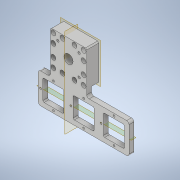
# Autodesk Inventor part: 30_XY_Sample_arm_UC2_Adapter_v3
Saved by Autodesk Inventor 2022.3 (Build 263350000, 350)
## iProperties
Created: 2020-12-29
Part Number: 30_XY_Sample_arm_UC2_Adapter_v3
Material: Generic
Document SubType Name: Modeling
Designer: diederichbenedict
Density: 1 g/cm^3
Appearance: Default
Author: diederichbenedict
Autodesk Inventor part; units mm, degrees
ref_plane "YZ Plane" through (0, 0, 0) normal (1, 0, 0) x (0, 1, 0)
ref_plane "XZ Plane" through (0, 0, 0) normal (0, 1, 0) x (-1, 0, 0)
ref_plane "XY Plane" through (0, 0, 0) normal (0, 0, 1) x (1, 0, 0)
ref_plane "Work Plane1" through (0, 0, 0) normal (0, 0, 1) x (1, 0, 0)
sketch "Sketch1" plane through (0, 0, 0) normal (0, 0, 1) x (1, 0, 0)
  circle A0 centre (-10, -25) radius 1.45 projected
  circle A1 centre (-10, 25) radius 1.45 projected
  circle A2 centre (10, 25) radius 1.45 projected
  circle A3 centre (10, -25) radius 1.45 projected
  circle A4 centre (-25, 25) radius 2.325 projected
  circle A5 centre (25, -25) radius 2.325 projected
  circle A6 centre (-25, -25) radius 2.325 projected
  circle A7 centre (25, 25) radius 2.325 projected
  line L0 (28, 30) -> (30, 28) projected
  line L1 (28, 30) -> (-28, 30) projected
  line L2 (-30, 28) -> (-28, 30) projected
  line L3 (-30, 28) -> (-30, -28) projected
  line L4 (-28, -30) -> (-30, -28) projected
  line L5 (-28, -30) -> (28, -30) projected
  line L6 (30, -28) -> (28, -30) projected
  line L7 (30, -28) -> (30, 28) projected
  circle A8 centre (-17.5, -17.5) radius 1.95 projected
  circle A9 centre (17.5, 17.5) radius 1.95 projected
  circle A10 centre (17.5, -17.5) radius 1.95 projected
  circle A11 centre (-17.5, 17.5) radius 1.95 projected
  circle A12 centre (0, 0) radius 7.5 projected
  circle A13 centre (-25.33, -75.26) radius 6.15 projected
  circle A14 centre (25, -10) radius 1.45 projected
  circle A15 centre (-25, -10) radius 1.45 projected
  circle A16 centre (-25, 10) radius 1.45 projected
  circle A17 centre (25, 10) radius 1.45 projected
  point P0 (0, 0)
extrude "Extrusion1" add sketch "Sketch1" along normal blind 12 contours L0 L7 L6 L5 L4 L3 L2 L1
sketch "Sketch2" plane through (0, 0, 12) normal (0, 0, 1) x (1, 0, 0)
  circle A0 centre (0, 0) radius 7.5 projected
  circle A1 centre (25, 10) radius 1.45 projected
  circle A2 centre (-25, 10) radius 1.45 projected
  circle A3 centre (-25, -10) radius 1.45 projected
  circle A4 centre (25, -10) radius 1.45 projected
  circle A5 centre (10, -25) radius 1.45 projected
  circle A6 centre (10, 25) radius 1.45 projected
  circle A7 centre (-10, 25) radius 1.45 projected
  circle A8 centre (-10, -25) radius 1.45 projected
  line L0 (-28, -30) -> (28, -30) projected
  line L1 (28, -30) -> (30, -28) projected
  line L2 (30, -28) -> (30, 28) projected
  line L3 (30, 28) -> (28, 30) projected
  line L4 (28, 30) -> (-28, 30) projected
  line L5 (30, -28) -> (30, 28) projected
  line L6 (30, -30) -> (28, -30)
  line L7 (18, -90) -> (30, -90)
  line L8 (30, -90) -> (30, -88) construction
  line L9 (30, 28) -> (30, -28) projected
  line L10 (30, -30) -> (30, -28)
  line L11 (30, -28) -> (28, -30)
  line L12 (-28, 30) -> (-30, 28) projected
  line L13 (-30, 28) -> (-30, -28) projected
  line L14 (-30, -28) -> (-28, -30) projected
  line L15 (-30, -30) -> (-28, -30)
  line L16 (-18, -90) -> (-30, -90)
  line L17 (-30, -30) -> (-30, -28)
  line L18 (-30, -28) -> (-28, -30)
  line L19 (-28, -30) -> (-30, -30)
  line L20 (28, -30) -> (30, -28) projected
  line L21 (28, -30) -> (30, -30)
  line L22 (30, -30) -> (30, -28)
  line L23 (30, -28) -> (28, -30)
  circle A9 centre (-17.5, 17.5) radius 1.95 projected
  circle A10 centre (-25, 25) radius 2.325 projected
  circle A11 centre (25, 25) radius 2.325 projected
  circle A12 centre (17.5, 17.5) radius 1.95 projected
  circle A13 centre (17.5, -17.5) radius 1.95 projected
  circle A14 centre (25, -25) radius 2.325 projected
  circle A15 centre (-25, -25) radius 2.325 projected
  line L24 (-18, -90) -> (18, -90)
  line L25 (18, -30) -> (-18, -30)
  line L26 (-50, -90) -> (-32, -90)
  line L27 (50, -90) -> (50, -40) construction
  line L28 (50, -40) -> (30, -40)
  line L29 (-50, -40) -> (-50, -90)
  line L30 (50, -40) -> (98, -40)
  line L31 (100, -40) -> (100, -42)
  line L32 (100, -90) -> (50, -90)
  line L33 (50, -90) -> (50, -40) construction
  line L34 (-30, -40) -> (-30, -30)
  line L35 (-30, -90) -> (-18, -90)
  line L36 (-18, -90) -> (18, -90)
  line L37 (18, -90) -> (30, -90)
  line L38 (30, -90) -> (32, -90)
  line L39 (32, -90) -> (50, -90)
  line L40 (100, -42) -> (100, -90)
  line L41 (98, -40) -> (100, -40)
  line L42 (30, -40) -> (18, -40)
  line L43 (-30, -90) -> (-30, -88) construction
  line L44 (-30, -40) -> (-50, -40)
  line L45 (-30, -88) -> (-30, -40) construction
  line L46 (-32, -90) -> (-30, -90)
  line L47 (18, -40) -> (-18, -40)
  line L48 (-18, -40) -> (-30, -40)
  line L49 (30, -40) -> (30, -30)
  line L50 (30, -88) -> (30, -40) construction
  line L51 (28, -30) -> (18, -30)
  line L52 (-28, -30) -> (-18, -30)
  line L53 (30, -28) -> (30, -30)
  line L54 (30, -28) -> (30, -30)
  line L55 (28, -30) -> (30, -30)
  line L56 (28, -30) -> (30, -28)
  point P0 (0, 0)
  point P1 (-24.2387, -104)
  point P2 (18, -80)
  point P3 (0, -40)
  point P4 (0, -30)
  dimension "d78" = 60
  dimension "d79" = 50
  dimension "d80" = 10
  dimension "d81" = 100
  dimension "d82" = 50
  constraints: 92 end point, 45 parallel, 14 horizontal, 13 collinear, 12 perpendicular, 12 point on line, 2 vertical, 1 midpoint, 1 vertical alignment
  measures "d78" distance between parallel lines of L0 L24
  measures "d79" distance between parallel lines of L26 L28
  measures "d80" distance from line of L28 L6.start
  measures "d81" distance between parallel lines of L27 L29
  measures "d82" distance between parallel lines of L31 L27
extrude "Extrusion2" add sketch "Sketch2" along normal blind 8
fillet "Fillet1" radius 4 6 edges at (-50, -40, 16) (-50, -90, 16) (100, -90, 16) (100, -40, 16) (30, -40, 16) (-30, -40, 16)
ref_plane "Work Plane2" through (-6, -91, 19) normal (1, 0, 0) x (0, 0, -1)
sketch "Sketch7" plane through (0, 0, 20) normal (0, 0, 1) x (1, 0, 0)
  circle A0 centre (10, -25) radius 1.45 projected
  circle A1 centre (-10, -25) radius 1.45 projected
  circle A2 centre (-25, -10) radius 1.45 projected
  circle A3 centre (-25, 10) radius 1.45 projected
  circle A4 centre (-10, 25) radius 1.45 projected
  circle A5 centre (10, 25) radius 1.45 projected
  circle A6 centre (25, 10) radius 1.45 projected
  circle A7 centre (25, -10) radius 1.45 projected
  circle A8 centre (-25, 25) radius 2.325 projected
  circle A9 centre (25, 25) radius 2.325 projected
  circle A10 centre (25, -25) radius 2.325 projected
  circle A11 centre (-25, -25) radius 2.325 projected
  point P0 (0, 0)
hole "Hole1" at (-25, -10, 20) at (-25, 10, 20) at (-10, 25, 20) at (10, 25, 20) at (25, 10, 20) at (25, -10, 20) at (10, -25, 20) at (-10, -25, 20) at (-25, 25, 20) at (-25, -25, 20) at (25, -25, 20) at (25, 25, 20) direction (0, 0, -1) diameter 3.2 end through all counterbore diameter 8 counterbore depth 10
sketch "Sketch12" plane through (0, 0, 12) normal (0, 0, -1) x (-1, 0, 0)
  line L0 (30.1502, -90.0017) -> (48, -90.0017)
  arc A0 (48, -90.0017) -> (50, -88.0017) centre (48, -88.0017) ccw
  line L1 (50, -70.0017) -> (50, -88.0017)
  arc A1 (50, -41.8579) -> (48, -39.8579) centre (48, -41.8579) ccw
  line L2 (48, -39.8579) -> (30, -39.8579)
  arc A2 (2, -40.0017) -> (0, -42.0017) centre (2, -42.0017) ccw
  line L3 (0, -59.8506) -> (0, -42.0017)
  arc A3 (0, -88.0017) -> (2, -90.0017) centre (2, -88.0017) ccw
  line L4 (9.561, -82.3) -> (40.161, -82.3)
  arc A4 (7.561, -80.3) -> (9.561, -82.3) centre (9.561, -80.3) ccw
  line L5 (7.561, -80.3) -> (7.561, -49.7)
  arc A5 (9.561, -47.7) -> (7.561, -49.7) centre (9.561, -49.7) ccw
  line L6 (40.161, -47.7) -> (9.561, -47.7)
  arc A6 (42.161, -49.7) -> (40.161, -47.7) centre (40.161, -49.7) ccw
  line L7 (42.161, -49.7) -> (42.161, -80.3)
  arc A7 (40.161, -82.3) -> (42.161, -80.3) centre (40.161, -80.3) ccw
  circle A8 centre (46.161, -65) radius 3.89
  circle A9 centre (24.761, -43.7) radius 2.9259
  line L8 (50, -70.0017) -> (50.8263, -70.0017)
  arc A10 (51.3, -70.3417) -> (50.8263, -70.0017) centre (50.8263, -70.5017) ccw
  arc A11 (51.3, -70.3417) -> (53.2596, -71.9417) centre (53.2596, -69.9417) ccw
  line L9 (53.2596, -71.9417) -> (53.4, -71.9417)
  arc A12 (53.4, -71.9417) -> (55.4, -69.9417) centre (53.4, -69.9417) ccw
  line L10 (55.4, -69.9417) -> (55.4, -60.0583)
  arc A13 (55.4, -60.0583) -> (53.4, -58.0583) centre (53.4, -60.0583) ccw
  line L11 (53.4, -58.0583) -> (53.2596, -58.0583)
  arc A14 (53.2596, -58.0583) -> (51.3, -59.6583) centre (53.2596, -60.0583) ccw
  arc A15 (50.8263, -59.9983) -> (51.3, -59.6583) centre (50.8263, -59.4983) ccw
  line L12 (50.8263, -59.9983) -> (50, -59.9983)
  line L13 (50, -41.8579) -> (50, -59.9983)
  line L14 (30, -39.8579) -> (30, -39.1754)
  arc A16 (30.34, -38.7017) -> (30, -39.1754) centre (30.5, -39.1754) ccw
  arc A17 (30.34, -38.7017) -> (31.94, -36.7421) centre (29.94, -36.7421) ccw
  line L15 (31.94, -36.7421) -> (31.94, -36.6017)
  arc A18 (31.94, -36.6017) -> (29.94, -34.6017) centre (29.94, -36.6017) ccw
  line L16 (29.94, -34.6017) -> (20.06, -34.6017)
  arc A19 (20.06, -34.6017) -> (18.06, -36.6017) centre (20.06, -36.6017) ccw
  line L17 (18.06, -36.6017) -> (18.06, -36.7421)
  arc A20 (18.06, -36.7421) -> (19.66, -38.7017) centre (20.06, -36.7421) ccw
  arc A21 (20, -39.1754) -> (19.66, -38.7017) centre (19.5, -39.1754) ccw
  line L18 (20, -39.1754) -> (20, -40.0017)
  line L19 (20, -40.0017) -> (2, -40.0017)
  line L20 (19.8489, -90.0017) -> (19.8491, -89.2759)
  arc A22 (19.8491, -89.2759) -> (19.6194, -88.9515) centre (19.5001, -89.2795) ccw
  arc A23 (17.9053, -86.8424) -> (19.6194, -88.9515) centre (20.06, -86.8424) ccw
  line L21 (17.9053, -86.8424) -> (17.9053, -86.7026)
  arc A24 (20.0566, -84.5515) -> (17.9053, -86.7026) centre (20.0565, -86.7026) ccw
  line L22 (20.0566, -84.5515) -> (29.94, -84.552)
  arc A25 (32.09, -86.7021) -> (29.94, -84.552) centre (29.94, -86.702) ccw
  line L23 (32.09, -86.7021) -> (32.09, -86.8424)
  arc A26 (30.38, -88.9468) -> (32.09, -86.8424) centre (29.9401, -86.8423) ccw
  arc A27 (30.38, -88.9468) -> (30.1502, -89.2756) centre (30.5004, -89.2756) ccw
  line L24 (30.1502, -89.2756) -> (30.1502, -90.0017)
  line L25 (0, -59.8506) -> (0.7258, -59.8508)
  arc A28 (0.7258, -59.8508) -> (1.0502, -59.6211) centre (0.7222, -59.5018) ccw
  arc A29 (3.1593, -57.907) -> (1.0502, -59.6211) centre (3.1593, -60.0617) ccw
  line L26 (3.1593, -57.907) -> (3.2991, -57.907)
  arc A30 (5.4502, -60.0583) -> (3.2991, -57.907) centre (3.2991, -60.0582) ccw
  line L27 (5.4502, -60.0583) -> (5.4497, -69.9417)
  arc A31 (3.2996, -72.0917) -> (5.4497, -69.9417) centre (3.2997, -69.9417) ccw
  line L28 (3.2996, -72.0917) -> (3.1593, -72.0917)
  arc A32 (1.0549, -70.3817) -> (3.1593, -72.0917) centre (3.1594, -69.9418) ccw
  arc A33 (1.0549, -70.3817) -> (0.7261, -70.1519) centre (0.7261, -70.5021) ccw
  line L29 (0.7261, -70.1519) -> (0, -70.152)
  line L30 (0, -88.0017) -> (0, -70.152)
  line L31 (2, -90.0017) -> (19.8489, -90.0017)
  line L32 (50, -44) -> (50, -86) projected
  line L33 (-0.1817, -64.8173) -> (24.3267, -108.886) construction
  line L34 (-100, -86) -> (-100, -44) projected
  line L35 (50, -44) -> (50, -86) projected
  point P0 (24.211, -65)
  point P1 (50, -65)
  point P2 (55.4, -65)
  point P3 (42.161, -65)
  point P4 (50, -65)
  point P5 (5.45, -65)
  point P6 (50, -65)
  point P7 (7.561, -65)
  point P8 (50, -65)
  point P9 (50, -65)
  dimension "d106" = 7.78
  dimension "d107" = 4
  dimension "d108" = 21.4
  dimension "d109" = 4
  constraints: 66 end point, 64 point on circle, 34 centre point, 7 horizontal alignment, 5 midpoint, 1 coincident, 1 collinear, 5 other
  measures "d106" diameter of A8
  measures "d107" distance from line of A8.centre L7
  measures "d108" horizontal distance of A9.centre A8.centre
  measures "d109" distance from line of L6 A9.centre
hole "Hole2" at (-46.161, -65, 12) at (-24.761, -43.7, 12) direction (0, 0, 1) diameter 3.2 end through all
pattern_linear "Rectangular Pattern1" count 3 spacing 50 along (1, 0, 0) of "Hole2"
sketch "Sketch15" plane through (0, 0, 12) normal (0, 0, -1) x (-1, 0, 0)
  line L0 (50, -40) -> (0, -40)
  line L1 (-100, -40) -> (-100, -90)
  line L2 (-100, -90) -> (-50, -90)
  line L3 (50, -90) -> (50, -40)
  line L4 (46, -90) -> (-96, -90) projected
  line L5 (-50, -40) -> (-50, -90)
  line L6 (50, -44) -> (50, -86) projected
  arc A0 (50, -44) -> (46, -40) centre (46, -44) ccw projected
  line L7 (34, -40) -> (46, -40) projected
  arc A1 (30, -36) -> (34, -40) centre (34, -36) ccw projected
  line L8 (30, -28) -> (30, -36) projected
  arc A2 (46, -90) -> (50, -86) centre (46, -86) ccw projected
  line L9 (46, -90) -> (-96, -90) projected
  arc A3 (-100, -86) -> (-96, -90) centre (-96, -86) ccw projected
  line L10 (-100, -86) -> (-100, -44) projected
  arc A4 (-96, -40) -> (-100, -44) centre (-96, -44) ccw projected
  line L11 (-96, -40) -> (-34, -40) projected
  arc A5 (-34, -40) -> (-30, -36) centre (-34, -36) ccw projected
  line L12 (-30, -36) -> (-30, -28) projected
  line L13 (0, -40) -> (0, -90)
  line L14 (42.3, -47.7) -> (7.7, -47.7)
  line L15 (7.7, -47.7) -> (7.7, -82.3)
  line L16 (7.7, -82.3) -> (42.3, -82.3)
  line L17 (42.3, -82.3) -> (42.3, -47.7)
  line L18 (-7.7, -47.7) -> (-42.3, -47.7)
  line L19 (-42.3, -47.7) -> (-42.3, -82.3)
  line L20 (-42.3, -82.3) -> (-7.7, -82.3)
  line L21 (-7.7, -82.3) -> (-7.7, -47.7)
  line L22 (-57.7, -47.7) -> (-92.3, -47.7)
  line L23 (-92.3, -47.7) -> (-92.3, -82.3)
  line L24 (-92.3, -82.3) -> (-57.7, -82.3)
  line L25 (-57.7, -82.3) -> (-57.7, -47.7)
  line L26 (0, -90) -> (50, -90)
  line L27 (-50, -90) -> (0, -90)
  line L28 (-50, -40) -> (-100, -40)
  line L29 (0, -40) -> (-50, -40)
  point P0 (0, 0)
  point P1 (0, -65)
  point P2 (42.3, -65)
  point P3 (50, -65)
  point P4 (-7.7, -65)
  point P5 (50, -65)
  point P6 (50, -65)
  point P7 (-57.7, -65)
  point P8 (25, -82.3)
  point P9 (25, -90)
  point P10 (-25, -82.3)
  point P11 (-25, -90)
  point P12 (-75, -82.3)
  point P13 (-75, -90)
  dimension "d116" = 50
  dimension "d117" = 50
  dimension "d118" = 50
  dimension "d119" = 34.6
  dimension "d120" = 34.6
  dimension "d121" = 34.6
  dimension "d122" = 34.6
  dimension "d123" = 34.6
  dimension "d124" = 34.6
  constraints: 44 end point, 16 parallel, 13 midpoint, 12 perpendicular, 8 collinear, 6 horizontal, 3 horizontal alignment, 3 point on line, 3 vertical alignment
  measures "d116" distance from line of point (0, -65) L3
  measures "d117" distance between parallel lines of L5 L1
  measures "d118" distance between parallel lines of L5 L13
  measures "d119" distance between parallel lines of L15 L17
  measures "d120" distance between parallel lines of L14 L16
  measures "d121" distance of L20.end L18.start
  measures "d122" distance between parallel lines of L19 L21
  measures "d123" distance of L24.end L22.start
  measures "d124" distance between parallel lines of L23 L25
extrude "Extrusion10" cut sketch "Sketch15" against normal blind 10 contours L17 L16 L15 L14 | L21 L20 L19 L18 | L25 L24 L23 L22
fillet "Fillet2" radius 2 12 edges at (-42.3, -82.3, 16) (-42.3, -47.7, 16) (-7.7, -47.7, 16) (42.3, -47.7, 16) (-7.7, -82.3, 16) (7.7, -47.7, 16) (7.7, -82.3, 16) (57.7, -82.3, 16) (42.3, -82.3, 16) (92.3, -82.3, 16) (57.7, -47.7, 16) (92.3, -47.7, 16)
ref_plane "Work Plane3" through (-46, -65, 12) normal (0, -1, 0) x (1, 0, 0)
mirror "Mirror2" about plane through (-46, -65, 12) normal (0, -1, 0) of "Hole2", "Rectangular Pattern1"
body "Solid1"
